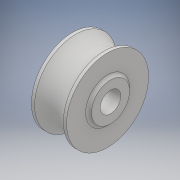
# Autodesk Inventor part: parte2_revolucion
Saved by Autodesk Inventor 2018 (Build 220112000, 112)
## iProperties
Created: 2018-04-06
Part Number: parte2_revolucion
Material: Generic
Document SubType Name: Modeling
Designer: Francisco
Density: 1 g/cm^3
Appearance: Default
Author: Francisco
Autodesk Inventor part; units mm, degrees
ref_plane "YZ Plane" through (0, 0, 0) normal (1, 0, 0) x (0, 1, 0)
ref_plane "XZ Plane" through (0, 0, 0) normal (0, 1, 0) x (-1, 0, 0)
ref_plane "XY Plane" through (0, 0, 0) normal (0, 0, 1) x (1, 0, 0)
sketch "Sketch1" plane through (0, 0, 0) normal (0, 0, 1) x (1, 0, 0)
  line L0 (-2, 7) -> (26, 7)
  line L1 (-13.8022, 0) -> (14.1978, 0) construction
  line L2 (26, 7) -> (26, 13)
  line L3 (26, 13) -> (24, 13)
  line L4 (24, 13) -> (24, 28)
  line L5 (0, 28) -> (0, 13)
  line L6 (0, 13) -> (-2, 13)
  line L7 (-2, 13) -> (-2, 7)
  arc A0 (2.202, 28) -> (21.798, 28) centre (12, 38) ccw
  arc A1 (2.202, 28) -> (21.798, 28) centre (12, 38) ccw
  line L8 (2.202, 28) -> (0, 28)
  line L9 (21.798, 28) -> (24, 28)
  point P0 (0, 0)
  dimension "d0" = 28
  dimension "d1" = 14
  dimension "d2" = 26
  dimension "d3" = 2
  dimension "d5" = 24
  dimension "d11" = 14
  dimension "d12" = 56
  dimension "d13" = 76
  constraints: 20 end point, 5 horizontal, 4 equal length, 4 point on circle, 2 centre point, 2 perpendicular, 2 point on line, 1 coincident, 1 vertical
  measures "d0" distance of L0.start L0.end
  measures "d1" diameter of L0 L1
  measures "d2" diameter of L2.end L1
  measures "d3" distance of L2.end L3.end
  measures "d5" distance between parallel lines of L4 L5
  measures "d11" radius of A1
  measures "d12" diameter of L9 L1
  measures "d13" diameter of A0.centre L1
revolve "Revolution1" add sketch "Sketch1" angle 360 about axis through (-13.8022, 0, 0) along (1, 0, 0)
fillet "Fillet1" radius 2 2 edges at (24, -13, 0) (0, -13, 0)
body "Solid1"
